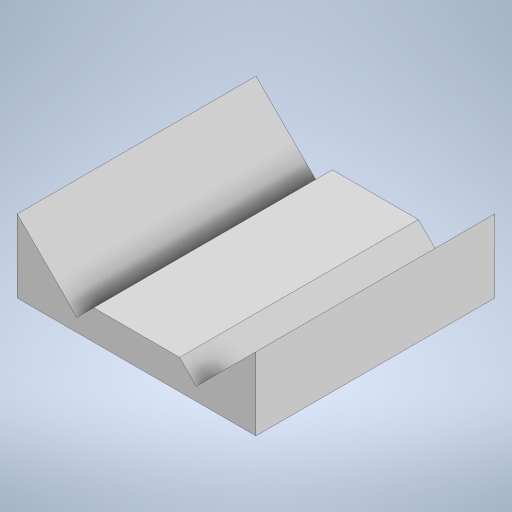
# Autodesk Inventor part: Drone Charging Base
Saved by Autodesk Inventor 2023 (Build 270158000, 158)
## iProperties
Created: 2022-12-15
Part Number: Drone Charging Base
Material: Generic
Document SubType Name: Modeling
Designer: chase
Density: 1 g/cm^3
Appearance: Default
Author: chase
Autodesk Inventor part; units mm, degrees
ref_plane "YZ Plane" through (0, 0, 0) normal (1, 0, 0) x (0, 1, 0)
ref_plane "XZ Plane" through (0, 0, 0) normal (0, 1, 0) x (-1, 0, 0)
ref_plane "XY Plane" through (0, 0, 0) normal (0, 0, 1) x (1, 0, 0)
sketch "Sketch1" plane through (0, 0, 0) normal (0, 0, 1) x (1, 0, 0)
  line L0 (0, 0) -> (914.4, 0)
  line L1 (914.4, 0) -> (914.4, 279.0857)
  line L2 (0, 279.0857) -> (0, 0)
  line L3 (685.8, 0) -> (685.8, 50.4857)
  line L4 (228.6, 0) -> (228.6, 50.4857)
  line L5 (228.6, 50.4857) -> (-130.6102, 409.6959)
  line L6 (685.8, 50.4857) -> (621.9857, 114.3)
  line L7 (685.8, 50.4857) -> (1045.0102, 409.6959)
  line L8 (330.2, 0) -> (330.2, 114.3)
  line L9 (127, 0) -> (127, 152.4)
  line L10 (584.2, 0) -> (584.2, 114.3)
  line L11 (787.4, 0) -> (787.4, 152.4)
  line L12 (228.6, 50.4857) -> (292.4143, 114.3)
  line L13 (330.2, 152.0857) -> (330.5143, 152.4)
  line L14 (127, 114.3) -> (126.6857, 114.3)
  line L15 (787.7143, 114.3) -> (787.4, 114.3)
  line L16 (621.9857, 114.3) -> (292.4143, 114.3)
  line L17 (787.7143, 152.4) -> (787.4, 152.4)
  line L18 (127, 152.4) -> (126.6857, 152.4)
  point P0 (583.8857, 152.4)
  point P1 (330.2, 152.4)
  point P2 (787.4, 152.0857)
  dimension "d18" = 101.6
  dimension "d19" = 101.6
  dimension "d20" = 101.6
  dimension "d21" = 101.6
  constraints: 38 end point, 13 parallel, 12 point on line, 1 horizontal, 1 perpendicular, 2 other
  measures "d18" distance between parallel lines of L4 L8
  measures "d19" distance between parallel lines of L4 L9
  measures "d20" distance between parallel lines of L3 L10
  measures "d21" distance between parallel lines of L3 L11
extrude "Extrusion1" add sketch "Sketch1" against normal blind 914.4 contours L2 L5 L9 L0 | L9 L5 L4 L0 | L4 L12 L16 L8 L0 | L8 L16 L10 L0 | L10 L16 L6 L3 L0 | L3 L7 L11 L0 | L11 L7 L1 L0
body "Solid1"
